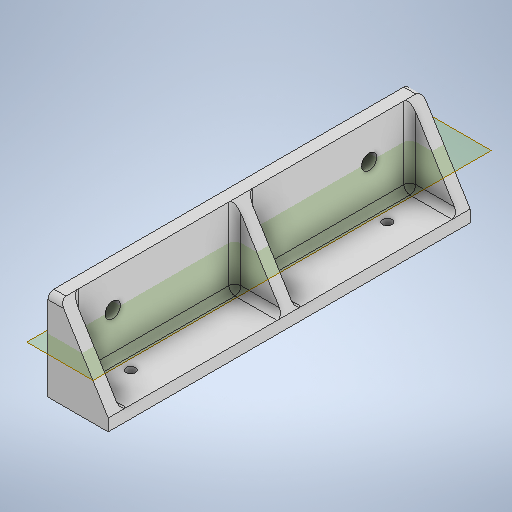
# Autodesk Inventor part: LV_Bracket
Saved by Autodesk Inventor 2025 (Build 290162000, 162)
## iProperties
Created: 2025-05-19
Part Number: LV_Bracket
Material: Generic
Document SubType Name: Modeling
Designer: mumin
Density: 1 g/cm^3
Appearance: Default
Author: mumin
Autodesk Inventor part; units mm, degrees
ref_plane "YZ Plane" through (0, 0, 0) normal (1, 0, 0) x (0, 1, 0)
ref_plane "XZ Plane" through (0, 0, 0) normal (0, 1, 0) x (-1, 0, 0)
ref_plane "XY Plane" through (0, 0, 0) normal (0, 0, 1) x (1, 0, 0)
sketch "Sketch1" plane through (0, 0, 0) normal (0, 0, 1) x (1, 0, 0)
  line L0 (-4, 26) -> (-4, -4)
  line L1 (-4, -4) -> (16, -4)
  line L2 (16, -4) -> (16, 0)
  line L3 (16, 0) -> (0, 0)
  line L4 (0, 0) -> (0, 26)
  line L5 (0, 26) -> (-4, 26)
  point P0 (0, 0)
  dimension "d0" = 30
  dimension "d1" = 20
  dimension "d2" = 4
  dimension "d3" = 4
  constraints: 12 end point, 5 perpendicular, 1 vertical
  measures "d0" distance of L0.start L0.end
  measures "d1" distance of L0.end L1.end
  measures "d2" distance of L1.end L2.end
  measures "d3" distance between parallel lines of L4 L0
extrude "Extrusion1" add sketch "Sketch1" along normal mid plane 120
sketch "Sketch2" plane through (0, 0, 0) normal (0, 0, 1) x (1, 0, 0)
  line L0 (0, 0) -> (0, 26) projected
  line L1 (16, -4) -> (16, 0) projected
  line L2 (0, 26) -> (16, 0)
  line L3 (16, 0) -> (0, 0)
  constraints: 4 end point, 1 perpendicular
extrude "Extrusion2" add sketch "Sketch2" along normal mid plane 4
pattern_linear "Rectangular Pattern1" count 3 spacing 58 along (0, 0, 1) of "Extrusion2" first direction both ways yes
fillet "Fillet1" radius 2 12 edges at (0, 0, 29) (0, 0, -29) (0, 13, 2) (8, 0, 2) (0, 13, -2) (8, 0, -2) (8, 0, 56) (0, 13, 56) (0, 13, -56) (8, 0, -56) (-2, 26, 60) (-2, 26, -60)
sketch "Sketch3" plane through (0, 2, 4) normal (1, 0, 0) x (0, 0, -1)
  line L0 (64, -6) -> (-56, -6) projected
  line L1 (8, 24) -> (0, 24) projected
  point P0 (4, -2)
  point P1 (-38.5, 12.28)
  point P2 (4, 24)
  dimension "d19" = 18.28
  dimension "d20" = 42.5
  constraints: 1 midpoint
  measures "d19" distance from line of L0 point (-38.5, 12.28)
  measures "d20" horizontal distance of point (4, 24) point (-38.5, 12.28)
hole "Hole1" at (0, 14.28, 42.5) direction (-1, 0, 0) diameter 5.1 depth 4 tip angle 118
mirror "Mirror1" about plane through (0, 0, 0) normal (0, 0, 1) of "Hole1"
sketch "Sketch4" plane through (2, 0, 4) normal (0, 1, 0) x (1, 0, 0)
  line L0 (14, 0) -> (14, -50) projected
  line L1 (14, 8) -> (14, 0) projected
  point P0 (-2, 4)
  point P1 (4, -38.5)
  point P2 (14, 4)
  dimension "d28" = 10
  dimension "d29" = 42.5
  constraints: 1 midpoint
  measures "d28" distance from line of L0 point (4, -38.5)
  measures "d29" vertical distance of point (14, 4) point (4, -38.5)
hole "Hole2" at (6, 0, 42.5) direction (0, -1, 0) diameter 3.1 depth 4 tip angle 118
mirror "Mirror2" about plane through (0, 0, 0) normal (0, 0, 1) of "Hole2"
ref_plane "Work Plane1" through (-4, 14.28, 60) normal (0, -1, 0) x (1, 0, 0)
sketch "Sketch5" plane through (-4, -4, -60) normal (-1, 0, 0) x (0, 0, 1)
  circle A0 centre (89, 18.28) radius 1.75
  line L0 (144, 18.28) -> (-24, 18.28) projected
  line L1 (120, 28) -> (120, 0) projected
  circle A1 centre (29.5, 18.28) radius 1.75
  circle A2 centre (17.5, 18.28) radius 2.55 projected
  point P0 (60, 4)
  dimension "d31" = 3.5
  dimension "d32" = 31
  dimension "d33" = 3.5
  dimension "d34" = 12
  constraints: 2 centre point, 2 point on line
  measures "d31" diameter of A0
  measures "d32" distance from line of L1 A0.centre
  measures "d33" diameter of A1
  measures "d34" distance of A1.centre A2.centre
extrude "Extrusion3" add sketch "Sketch5" along normal blind 3 contours L0 A0 | A0 L0 | A1 L0 | L0 A1
fillet "Fillet2" radius 1 2 edges at (-7, 14.28, -32.25) (-7, 14.28, 27.25)
body "Solid1"
